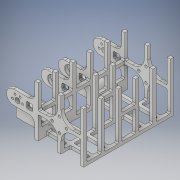
# Autodesk Inventor part: Double Holder V5
Saved by Autodesk Inventor 2019 (Build 230136000, 136)
## iProperties
Created: 2018-12-02
Part Number: Double Holder V5
Material: Generic
Document SubType Name: Modeling
Designer: Ashley
Density: 1 g/cm^3
Appearance: Default
Author: Ashley
Autodesk Inventor part; units mm, degrees
ref_plane "YZ Plane" through (0, 0, 0) normal (1, 0, 0) x (0, 1, 0)
ref_plane "XZ Plane" through (0, 0, 0) normal (0, 1, 0) x (-1, 0, 0)
ref_plane "XY Plane" through (0, 0, 0) normal (0, 0, 1) x (1, 0, 0)
sketch "Sketch1" plane through (0, 0, 0) normal (0, 1, 0) x (-1, 0, 0)
  line L0 (-40.25, -64) -> (40.25, -64) construction
  line L1 (40.25, -64) -> (40.25, 64) construction
  line L2 (40.25, 64) -> (-40.25, 64) construction
  line L3 (-40.25, 64) -> (-40.25, -64) construction
  line L4 (-40.25, -64) -> (40.25, 64) construction
  line L5 (40.25, -64) -> (-40.25, 64) construction
  line L6 (38.5, 71) -> (-38.5, 71) construction
  line L7 (-38.5, 71) -> (-38.5, 11) construction
  line L8 (-38.5, 11) -> (38.5, 11) construction
  line L9 (38.5, 11) -> (38.5, 71) construction
  line L10 (49.194, 0) -> (-57.7612, 0) construction
  line L11 (38.5, -71) -> (-38.5, -71) construction
  line L12 (-38.5, -71) -> (-38.5, -11) construction
  line L13 (-38.5, -11) -> (38.5, -11) construction
  line L14 (38.5, -11) -> (38.5, -71) construction
  line L15 (-38.5, -21) -> (-38.5, -31)
  line L16 (38.5, -31) -> (38.5, -21)
  line L17 (-38.5, -41) -> (-38.5, -51)
  line L18 (38.5, -51) -> (38.5, -41)
  line L19 (-38.5, 21) -> (-38.5, 31)
  line L20 (38.5, 31) -> (38.5, 21)
  line L21 (-38.5, 41) -> (-38.5, 51)
  line L22 (38.5, 51) -> (38.5, 41)
  line L23 (38.5, -11) -> (33.5, -11)
  line L24 (33.5, -71) -> (38.5, -71)
  line L25 (38.5, -71) -> (38.5, -11)
  line L26 (-38.5, -71) -> (-33.5, -71)
  line L27 (-33.5, -11) -> (-38.5, -11)
  line L28 (-38.5, -11) -> (-38.5, -71)
  line L29 (-38.5, 71) -> (-38.5, 11) construction
  line L30 (38.5, 11) -> (38.5, 71) construction
  line L31 (-38.5, 21) -> (-38.5, 31)
  line L32 (38.5, 31) -> (38.5, 21)
  line L33 (-38.5, 41) -> (-38.5, 51)
  line L34 (38.5, 51) -> (38.5, 41)
  line L35 (38.5, 11) -> (33.5, 11)
  line L36 (33.5, 71) -> (38.5, 71)
  line L37 (38.5, 71) -> (38.5, 11)
  line L38 (-38.5, 71) -> (-33.5, 71)
  line L39 (-33.5, 11) -> (-38.5, 11)
  line L40 (-38.5, 11) -> (-38.5, 71)
  line L41 (33.5, 11) -> (33.5, 26)
  line L42 (33.5, 31) -> (33.5, 51)
  line L43 (33.5, 56) -> (33.5, 71)
  line L44 (-33.5, 71) -> (-33.5, 56)
  line L45 (-33.5, 26) -> (-33.5, 11)
  line L46 (33.5, -11) -> (33.5, -26)
  line L47 (33.5, -31) -> (33.5, -51)
  line L48 (33.5, -56) -> (33.5, -71)
  line L49 (-33.5, -71) -> (-33.5, -56)
  line L50 (-33.5, -51) -> (-33.5, -31)
  line L51 (-33.5, -26) -> (-33.5, -11)
  line L52 (-33.5, 51) -> (-33.5, 31)
  line L53 (-2.5, -71) -> (2.5, -71)
  line L54 (2.5, 71) -> (-2.5, 71)
  line L55 (-2.5, -71) -> (2.5, 71) construction
  line L56 (2.5, -71) -> (-2.5, 71) construction
  line L57 (2.5, 56) -> (2.5, 71)
  line L58 (-33.5, 56) -> (-2.5, 56)
  line L59 (2.5, 56) -> (33.5, 56)
  line L60 (-2.5, 71) -> (-2.5, 56)
  line L61 (33.5, 51) -> (2.5, 51)
  line L62 (-2.5, 51) -> (-33.5, 51)
  line L63 (2.5, 31) -> (2.5, 51)
  line L64 (-33.5, 31) -> (-2.5, 31)
  line L65 (2.5, 31) -> (33.5, 31)
  line L66 (33.5, 26) -> (2.5, 26)
  line L67 (-2.5, 26) -> (-33.5, 26)
  line L68 (-2.5, 51) -> (-2.5, 31)
  line L69 (2.5, -26) -> (2.5, 26)
  line L70 (33.5, -26) -> (2.5, -26)
  line L71 (-2.5, -26) -> (-33.5, -26)
  line L72 (-33.5, -31) -> (-2.5, -31)
  line L73 (2.5, -31) -> (33.5, -31)
  line L74 (-2.5, 26) -> (-2.5, -26)
  line L75 (2.5, -71) -> (2.5, -56)
  line L76 (2.5, -51) -> (2.5, -31)
  line L77 (33.5, -51) -> (2.5, -51)
  line L78 (-2.5, -51) -> (-33.5, -51)
  line L79 (-33.5, -56) -> (-2.5, -56)
  line L80 (2.5, -56) -> (33.5, -56)
  line L81 (-2.5, -31) -> (-2.5, -51)
  line L82 (-2.5, -56) -> (-2.5, -71)
  point P0 (0, 0)
  dimension "d219" = 0
  dimension "d0" = 128
  dimension "d6" = 11
  dimension "d7" = 60
  dimension "d31" = 5
  dimension "d32" = 5
  dimension "d33" = 5
  dimension "d34" = 5
  dimension "d35" = 5
  dimension "d37" = 5
  dimension "d38" = 5
  dimension "d39" = 5
  dimension "d52" = 5
  dimension "d328" = 60
  dimension "d329" = 20
  dimension "d330" = 15
  dimension "d332" = 5
  dimension "d333" = 5
  dimension "d334" = 15
  dimension "d335" = 15
  dimension "d337" = 20
  dimension "d343" = 15
  dimension "d344" = 5
  dimension "d345" = 5
  dimension "d359" = 5
  dimension "d360" = 20
  dimension "d361" = 15
  dimension "d362" = 0
  dimension "d363" = 15
  dimension "d364" = 20
  dimension "d365" = 15
  dimension "d366" = 5
  dimension "d367" = 5
  dimension "d368" = 5
  dimension "d369" = 15
  dimension "d394" = 31
  dimension "d398" = 80.5
  dimension "d400" = 77
  dimension "d401" = 31
  dimension "d402" = 31
  dimension "d403" = 31
  dimension "d441" = 31
  dimension "d442" = 31
  dimension "d443" = 31
  dimension "d444" = 31
  dimension "d445" = 31
  dimension "d446" = 31
  dimension "d447" = 31
  dimension "d448" = 31
  constraints: 166 end point, 48 parallel, 20 symmetric about line, 19 perpendicular, 11 horizontal, 8 point on line, 6 midpoint
  measures "d0" distance of L0.end L1.end
  measures "d6" distance between parallel lines of L10 L8
  measures "d7" distance of L8.end L6.start
  measures "d31" distance between parallel lines of L9 L41
  measures "d32" distance between parallel lines of L9 L42
  measures "d33" distance between parallel lines of L9 L43
  measures "d34" distance between parallel lines of L14 L47
  measures "d35" distance between parallel lines of L12 L50
  measures "d37" distance between parallel lines of L7 L45
  measures "d38" distance between parallel lines of L7 L52
  measures "d39" distance between parallel lines of L7 L44
  measures "d52" distance of L54.end L54.start
  measures "d328" distance of L13.end L11.start
  measures "d329" distance between parallel lines of L62 L64
  measures "d330" distance between parallel lines of L67 L8
  measures "d332" distance between parallel lines of L58 L62
  measures "d333" distance between parallel lines of L64 L67
  measures "d334" distance between parallel lines of L6 L58
  measures "d335" distance between parallel lines of L8 L66
  measures "d337" distance between parallel lines of L61 L65
  measures "d343" distance between parallel lines of L6 L59
  measures "d344" distance between parallel lines of L65 L66
  measures "d345" distance between parallel lines of L59 L61
  measures "d359" distance between parallel lines of L77 L80
  measures "d360" distance between parallel lines of L73 L77
  measures "d361" distance between parallel lines of L11 L79
  measures "d362" distance between parallel lines of L11 L53
  measures "d363" distance between parallel lines of L11 L80
  measures "d364" distance between parallel lines of L72 L78
  measures "d365" distance between parallel lines of L13 L71
  measures "d366" distance between parallel lines of L79 L78
  measures "d367" distance between parallel lines of L70 L73
  measures "d368" distance between parallel lines of L71 L72
  measures "d369" distance between parallel lines of L13 L70
  measures "d394" distance between parallel lines of L63 L42
  measures "d398" distance between parallel lines of L3 L1
  measures "d400" distance between parallel lines of L9 L7
  measures "d401" distance between parallel lines of L68 L52
  measures "d402" distance between parallel lines of L81 L50
  measures "d403" distance between parallel lines of L47 L76
  measures "d441" distance between parallel lines of L43 L57
  measures "d442" distance between parallel lines of L44 L60
  measures "d443" distance between parallel lines of L69 L41
  measures "d444" distance between parallel lines of L45 L74
  measures "d445" distance between parallel lines of L46 L69
  measures "d446" distance between parallel lines of L51 L74
  measures "d447" distance between parallel lines of L75 L48
  measures "d448" distance between parallel lines of L49 L82
extrude "Base Extrusion" add sketch "Sketch1" along normal blind 5
sketch "Sketch4" plane through (0, 5, 0) normal (0, 1, 0) x (1, 0, 0)
  line L0 (-38.5, -71) -> (-33.5, -71)
  line L1 (-33.5, -71) -> (-33.5, -66)
  line L2 (-33.5, -66) -> (-38.5, -66)
  line L3 (-38.5, -66) -> (-38.5, -71)
  line L4 (-33.5, -11) -> (-38.5, -11)
  line L5 (-38.5, -11) -> (-38.5, -16)
  line L6 (-38.5, -16) -> (-33.5, -16)
  line L7 (-33.5, -16) -> (-33.5, -11)
  line L8 (2.5, -71) -> (-2.5, -71)
  line L9 (-2.5, -71) -> (-2.5, -66)
  line L10 (-2.5, -66) -> (2.5, -66)
  line L11 (2.5, -66) -> (2.5, -71)
  line L12 (33.5, -71) -> (38.5, -71)
  line L13 (38.5, -71) -> (38.5, -66)
  line L14 (38.5, -66) -> (33.5, -66)
  line L15 (33.5, -66) -> (33.5, -71)
  line L16 (38.5, -11) -> (33.5, -11)
  line L17 (33.5, -11) -> (33.5, -16)
  line L18 (33.5, -16) -> (38.5, -16)
  line L19 (38.5, -16) -> (38.5, -11)
  line L20 (38.5, -38.5) -> (33.5, -38.5)
  line L21 (33.5, -38.5) -> (33.5, -43.5)
  line L22 (33.5, -43.5) -> (38.5, -43.5)
  line L23 (38.5, -43.5) -> (38.5, -38.5)
  line L24 (38.5, -38.5) -> (33.5, -43.5) construction
  line L25 (33.5, -38.5) -> (38.5, -43.5) construction
  line L26 (2.5, -16) -> (-2.5, -16)
  line L27 (-2.5, -16) -> (-2.5, -11)
  line L28 (-2.5, -11) -> (2.5, -11)
  line L29 (2.5, -11) -> (2.5, -16)
  line L30 (2.5, -16) -> (-2.5, -11) construction
  line L31 (-2.5, -16) -> (2.5, -11) construction
  line L32 (-50.9334, 0) -> (57.8968, 0) construction
  line L33 (33.5, 71) -> (38.5, 71) construction
  line L34 (38.5, 11) -> (33.5, 11) construction
  line L35 (-33.5, 11) -> (-38.5, 11) construction
  line L36 (-38.5, 71) -> (-33.5, 71) construction
  line L37 (-38.5, 71) -> (-33.5, 71)
  line L38 (-33.5, 71) -> (-33.5, 66)
  line L39 (-33.5, 66) -> (-38.5, 66)
  line L40 (-38.5, 66) -> (-38.5, 71)
  line L41 (-33.5, 11) -> (-38.5, 11)
  line L42 (-38.5, 11) -> (-38.5, 16)
  line L43 (-38.5, 16) -> (-33.5, 16)
  line L44 (-33.5, 16) -> (-33.5, 11)
  line L45 (33.5, 71) -> (38.5, 71)
  line L46 (38.5, 71) -> (38.5, 66)
  line L47 (38.5, 66) -> (33.5, 66)
  line L48 (33.5, 66) -> (33.5, 71)
  line L49 (38.5, 11) -> (33.5, 11)
  line L50 (33.5, 11) -> (33.5, 16)
  line L51 (33.5, 16) -> (38.5, 16)
  line L52 (38.5, 16) -> (38.5, 11)
  line L53 (38.5, 38.5) -> (33.5, 38.5)
  line L54 (33.5, 38.5) -> (33.5, 43.5)
  line L55 (33.5, 43.5) -> (38.5, 43.5)
  line L56 (38.5, 43.5) -> (38.5, 38.5)
  line L57 (38.5, 38.5) -> (33.5, 43.5) construction
  line L58 (33.5, 38.5) -> (38.5, 43.5) construction
  line L59 (2.5, 16) -> (-2.5, 16)
  line L60 (-2.5, 16) -> (-2.5, 11)
  line L61 (-2.5, 11) -> (2.5, 11)
  line L62 (2.5, 11) -> (2.5, 16)
  line L63 (2.5, 16) -> (-2.5, 11) construction
  line L64 (-2.5, 16) -> (2.5, 11) construction
  line L65 (-33.5, 51) -> (-33.5, 31) construction
  line L66 (-38.5, 38.5) -> (-33.5, 38.5)
  line L67 (-33.5, 38.5) -> (-33.5, 43.5)
  line L68 (-33.5, 43.5) -> (-38.5, 43.5)
  line L69 (-38.5, 43.5) -> (-38.5, 38.5)
  line L70 (-38.5, 38.5) -> (-33.5, 43.5) construction
  line L71 (-33.5, 38.5) -> (-38.5, 43.5) construction
  line L72 (-38.5, -43.5) -> (-33.5, -43.5)
  line L73 (-33.5, -43.5) -> (-33.5, -38.5)
  line L74 (-33.5, -38.5) -> (-38.5, -38.5)
  line L75 (-38.5, -38.5) -> (-38.5, -43.5)
  line L76 (-38.5, -43.5) -> (-33.5, -38.5) construction
  line L77 (-33.5, -43.5) -> (-38.5, -38.5) construction
  line L78 (38.5, 71) -> (33.5, 71) construction
  line L79 (2.5, -71) -> (2.5, -56) construction
  line L80 (-2.5, 71) -> (2.5, 71)
  line L81 (2.5, 71) -> (2.5, 66)
  line L82 (2.5, 66) -> (-2.5, 66)
  line L83 (-2.5, 66) -> (-2.5, 71)
  line L84 (38.5, 11) -> (38.5, 71) construction
  line L85 (2.5, 56) -> (2.5, 71) construction
  line L86 (-33.5, -26) -> (-33.5, -11) construction
  line L87 (-38.5, -11) -> (-38.5, -71) construction
  point P0 (38.5, -71)
  point P1 (33.5, -11)
  point P2 (0, 0)
  point P3 (36, -41)
  point P4 (0, -13.5)
  point P5 (36, 41)
  point P6 (0, 13.5)
  point P7 (-36, 41)
  point P8 (-36, -41)
  dimension "d55" = 5
  dimension "d56" = 5
  dimension "d58" = 5
  dimension "d90" = 5
  dimension "d91" = 5
  dimension "d92" = 5
  dimension "d370" = 22.5
  dimension "d371" = 60
  dimension "d372" = 5
  dimension "d373" = 5
  dimension "d375" = 22.5
  dimension "d376" = 0
  dimension "d377" = 60
  dimension "d378" = 22.5
  dimension "d379" = 22.5
  dimension "d381" = 22.5
  dimension "d385" = 5
  dimension "d388" = 5
  dimension "d389" = 5
  dimension "d451" = 5
  dimension "d452" = 0
  dimension "d453" = 5
  dimension "d454" = 5
  dimension "d455" = 5
  dimension "d456" = 0
  dimension "d457" = 0
  dimension "d458" = 5
  dimension "d459" = 5
  dimension "d460" = 5
  dimension "d461" = 22.5
  dimension "d463" = 60
  dimension "d464" = 22.5
  dimension "d465" = 22.5
  constraints: 162 end point, 30 symmetric about line, 20 parallel, 12 midpoint, 11 horizontal, 10 perpendicular, 2 point on line
  measures "d55" distance of L1.end L0.end
  measures "d56" distance of L5.end L4.end
  measures "d58" distance of L21.end L20.end
  measures "d90" distance of L67.end L66.end
  measures "d91" distance of L74.end L73.end
  measures "d92" distance of L73.end L72.end
  measures "d370" distance between parallel lines of L51 L53
  measures "d371" distance between parallel lines of L34 L33
  measures "d372" distance between parallel lines of L53 L55
  measures "d373" distance between parallel lines of L47 L33
  measures "d375" distance between parallel lines of L47 L55
  measures "d376" distance between parallel lines of L45 L78
  measures "d377" distance of point (38.5, -71) L16.start
  measures "d378" distance between parallel lines of L14 L22
  measures "d379" distance between parallel lines of L20 L18
  measures "d381" distance between parallel lines of L39 L68
  measures "d385" distance between parallel lines of L9 L79
  measures "d388" distance of L81.end L82.end
  measures "d389" distance of L80.end L81.end
  measures "d451" distance between parallel lines of L48 L46
  measures "d452" distance between parallel lines of L84 L56
  measures "d453" distance between parallel lines of L54 L84
  measures "d454" distance between parallel lines of L52 L50
  measures "d455" distance between parallel lines of L34 L51
  measures "d456" distance between parallel lines of L85 L81
  measures "d457" distance between parallel lines of L87 L75
  measures "d458" distance between parallel lines of L3 L1
  measures "d459" distance between parallel lines of L86 L5
  measures "d460" distance between parallel lines of L67 L69
  measures "d461" distance between parallel lines of L43 L66
  measures "d463" distance of L87.start L0.start
  measures "d464" distance between parallel lines of L74 L6
  measures "d465" distance between parallel lines of L2 L72
extrude "Pegs Extrusions" add sketch "Sketch4" along normal blind 74.5
sketch "Sketch8" plane through (0, 5, 0) normal (0, 1, 0) x (1, 0, 0)
  line L0 (-38.5, 11) -> (-38.5, 71) construction
  line L1 (-33.5, 66) -> (-38.5, 66)
  line L2 (-38.5, 66) -> (-38.5, 16)
  line L3 (-38.5, 16) -> (-33.5, 16)
  line L4 (-33.5, 16) -> (-33.5, 66)
  line L5 (-38.5, -71) -> (-38.5, -11) construction
  line L6 (-38.5, -16) -> (-33.5, -16)
  line L7 (-33.5, -16) -> (-33.5, -66)
  line L8 (-33.5, -66) -> (-38.5, -66)
  line L9 (-38.5, -66) -> (-38.5, -16)
  line L10 (-33.5, -16) -> (-38.5, -16) projected
  line L11 (-38.5, -66) -> (-33.5, -66) projected
  line L12 (-33.5, 16) -> (-38.5, 16) construction
  line L13 (-38.5, 66) -> (-33.5, 66) construction
  point P0 (0, 0)
  dimension "d286" = 50
  dimension "d287" = 50
  dimension "d288" = 0
  dimension "d289" = 50
  dimension "d290" = 50
  dimension "d291" = 0
  dimension "d449" = 5
  dimension "d450" = 5
  constraints: 16 end point, 4 parallel, 2 horizontal, 2 perpendicular, 2 point on line
  measures "d286" distance between parallel lines of L8 L6
  measures "d287" distance between parallel lines of L11 L10
  measures "d288" distance between parallel lines of L6 L10
  measures "d289" distance between parallel lines of L12 L13
  measures "d290" distance between parallel lines of L3 L1
  measures "d291" distance between parallel lines of L13 L1
  measures "d449" distance between parallel lines of L0 L4
  measures "d450" distance between parallel lines of L5 L7
extrude "Front Extrusion" add sketch "Sketch8" along normal blind 11.5
sketch "Sketch9" plane through (-38.5, 0, 11) normal (-1, 0, 0) x (0, 0, 1)
  line L0 (11.5, 5) -> (48.5, 5) construction
  line L1 (8.0687, 8.5) -> (51.7383, 8.5) construction
  line L2 (9.6976, 12.5) -> (51.7383, 12.5) construction
  line L3 (43.5, 23.1119) -> (43.5, 2.014) construction
  line L4 (16.5, 23.1119) -> (16.5, 2.014) construction
  arc A0 (16.5, 12.5629) -> (43.5, 12.5629) centre (30, 32.9598) ccw
  line L5 (16.5, 12.5629) -> (16.5, 14.5629)
  line L6 (43.5, 12.5629) -> (43.5, 14.5629)
  arc A1 (16.5, 14.5629) -> (43.5, 14.5629) centre (30, 32.9598) ccw
  line L7 (60, 0) -> (60, 79.5) construction
  line L8 (-82, 0) -> (-82, 79.5) construction
  line L9 (32.5, 16.5) -> (32.5, 79.5) construction
  line L10 (27.5, 16.5) -> (27.5, 79.5) construction
  line L11 (5, 16.5) -> (5, 79.5) construction
  line L12 (55, 16.5) -> (55, 79.5) construction
  line L13 (0, 0) -> (0, 79.5) construction
  line L14 (-22, 0) -> (-22, 79.5) construction
  line L15 (-11, -14.5349) -> (-11, 42.196) construction
  line L16 (-33.5, 5) -> (-70.5, 5) construction
  line L17 (-30.0687, 8.5) -> (-73.7383, 8.5) construction
  line L18 (-31.6976, 12.5) -> (-73.7383, 12.5) construction
  line L19 (-65.5, 23.1119) -> (-65.5, 2.014) construction
  line L20 (-38.5, 23.1119) -> (-38.5, 2.014) construction
  arc A2 (-65.5, 12.5629) -> (-38.5, 12.5629) centre (-52, 32.9598) ccw
  line L21 (-38.5, 12.5629) -> (-38.5, 14.5629)
  line L22 (-65.5, 12.5629) -> (-65.5, 14.5629)
  arc A3 (-65.5, 14.5629) -> (-38.5, 14.5629) centre (-52, 32.9598) ccw
  dimension "d77" = 3.5
  dimension "d78" = 4
  dimension "d81" = 27
  dimension "d84" = 2
  dimension "d85" = 2
  dimension "d341" = 2.5
  dimension "d342" = 2.5
  dimension "d347" = 11.5
  dimension "d349" = 50
  dimension "d350" = 11.5
  dimension "d404" = 22
  dimension "d406" = 11
  constraints: 30 end point, 16 symmetric about line, 8 point on circle, 4 centre point, 4 point on line, 2 coincident, 2 horizontal, 2 midpoint, 2 vertical, 1 tangent, 2 other
  measures "d77" distance between parallel lines of L0 L1
  measures "d78" distance between parallel lines of L1 L2
  measures "d81" distance between parallel lines of L3 L4
  measures "d84" distance of L5.start L5.end
  measures "d85" distance of L6.start L6.end
  measures "d341" distance from line of A0.centre L10
  measures "d342" distance from line of L9 A0.centre
  measures "d347" distance between parallel lines of L4 L11
  measures "d349" distance between parallel lines of L12 L11
  measures "d350" distance between parallel lines of L12 L3
  measures "d404" distance between parallel lines of L13 L14
  measures "d406" distance between parallel lines of L13 L15
extrude "Tape MEasure Holes Sketch" cut sketch "Sketch9" against normal up to surface (5 mm away)
fillet "Fillet1" radius 0.5 2 edges at (-36, 14.5629, 27.5) (-36, 14.5629, 54.5)
fillet "Fillet2" radius 0.6 2 edges at (-36, 12.5629, 54.5) (-36, 12.5629, 27.5)
sketch "Sketch13" plane through (33.5, 0, 56) normal (-1, 0, 0) x (0, 0, 1)
  line L0 (15, 0) -> (0, 0) construction
  line L1 (10, 5) -> (10, 79.5) construction
  line L2 (10, 36.463) -> (15, 36.463)
  line L3 (15, 36.463) -> (15, 41.463)
  line L4 (15, 41.463) -> (10, 41.463)
  line L5 (10, 41.463) -> (10, 36.463)
  line L6 (-56, -4.0321) -> (-56, 65.3237) construction
  line L7 (-127, 0) -> (-127, 79.5) construction
  line L8 (-122, 5) -> (-122, 79.5) construction
  line L9 (-122, 36.463) -> (-127, 36.463)
  line L10 (-127, 36.463) -> (-127, 41.463)
  line L11 (-127, 41.463) -> (-122, 41.463)
  line L12 (-122, 41.463) -> (-122, 36.463)
  line L13 (-127, 0) -> (-127, 79.5) construction
  point P0 (15, 79.5)
  point P1 (-56, 0)
  dimension "d198" = 5
  dimension "d199" = 5
  dimension "d200" = 36.463
  dimension "d358" = 0
  constraints: 22 end point, 8 symmetric about line, 2 parallel, 2 point on line, 1 horizontal, 1 perpendicular, 1 vertical
  measures "d198" distance of L2.start L2.end
  measures "d199" distance between parallel lines of L2 L4
  measures "d200" distance between parallel lines of L0 L2
  measures "d358" distance between parallel lines of L13 L7
extrude "Side Reenforcements" add sketch "Sketch13" along normal blind 69.5
sketch "Sketch14" plane through (-38.5, 0, -71) normal (-1, 0, 0) x (0, 0, 1)
  line L0 (5, 16.5) -> (5, 79.5) construction
  line L1 (0, 0) -> (0, 79.5) construction
  line L2 (0, 51.663) -> (5, 51.663)
  line L3 (5, 51.663) -> (5, 29.463)
  line L4 (5, 29.463) -> (0, 29.463)
  line L5 (0, 29.463) -> (0, 51.663)
  line L6 (5, 41.463) -> (0, 41.463) construction
  line L7 (0, 41.463) -> (5, 41.463) construction
  line L8 (0, 36.463) -> (5, 36.463) construction
  line L9 (0, 36.463) -> (5, 36.463) construction
  line L10 (71, -9.8248) -> (71, 90.7022) construction
  line L11 (112, 28.863) -> (112, 84.0441) construction
  line L12 (-56, 28.863) -> (-56, 84.0441) construction
  arc A0 (16.5, 14.5629) -> (43.5, 14.5629) centre (30, 32.9598) ccw construction
  arc A1 (16.5, 12.5629) -> (43.5, 12.5629) centre (30, 32.9598) ccw construction
  line L13 (30, -7.2644) -> (30, 95.9334) construction
  line L14 (32.5, 16.5) -> (32.5, 79.5) construction
  line L15 (27.5, 16.5) -> (27.5, 79.5) construction
  line L16 (137, 16.5) -> (137, 79.5) construction
  line L17 (-11, -9.8248) -> (-11, 90.7022) construction
  line L18 (142, 51.663) -> (137, 51.663)
  line L19 (137, 51.663) -> (137, 29.463)
  line L20 (137, 29.463) -> (142, 29.463)
  line L21 (142, 29.463) -> (142, 51.663)
  line L22 (137, 41.463) -> (142, 41.463) construction
  line L23 (142, 41.463) -> (137, 41.463) construction
  line L24 (142, 36.463) -> (137, 36.463) construction
  line L25 (142, 36.463) -> (137, 36.463) construction
  line L26 (0, 79.5) -> (5, 79.5) construction
  line L27 (60, 0) -> (0, 0) construction
  line L28 (55, 79.5) -> (60, 79.5) construction
  line L29 (55, 5) -> (55, 79.5) construction
  line L30 (60, 0) -> (60, 79.5) construction
  line L31 (55, 49.663) -> (60, 49.663)
  line L32 (60, 49.663) -> (60, 28.263)
  line L33 (60, 28.263) -> (55, 28.263)
  line L34 (55, 28.263) -> (55, 49.663)
  line L35 (87, 5) -> (87, 79.5) construction
  line L36 (82, 0) -> (82, 79.5) construction
  line L37 (87, 49.663) -> (82, 49.663)
  line L38 (82, 49.663) -> (82, 28.263)
  line L39 (82, 28.263) -> (87, 28.263)
  line L40 (87, 28.263) -> (87, 49.663)
  point P0 (112, 32.9598)
  point P1 (112, 32.9598)
  dimension "d204" = 7
  dimension "d323" = 22.2
  dimension "d326" = 10.2
  dimension "d408" = 5
  dimension "d409" = 2.5
  dimension "d417" = 27.837
  dimension "d418" = 29.463
  dimension "d419" = 21.4
  dimension "d420" = 29.837
  dimension "d421" = 28.263
  constraints: 58 end point, 21 symmetric about line, 7 point on line, 4 parallel, 3 perpendicular, 2 horizontal, 2 vertical
  measures "d204" distance between parallel lines of L4 L8
  measures "d323" distance between parallel lines of L4 L2
  measures "d326" distance between parallel lines of L6 L2
  measures "d408" distance between parallel lines of L14 L15
  measures "d409" distance between parallel lines of L14 L13
  measures "d417" distance between parallel lines of L26 L2
  measures "d418" distance between parallel lines of L27 L4
  measures "d419" distance between parallel lines of L33 L31
  measures "d420" distance between parallel lines of L28 L31
  measures "d421" distance between parallel lines of L27 L33
extrude "Siding Extrusions" add sketch "Sketch14" along normal blind 45.1
sketch "Sketch17" plane through (38.5, 0, -71) normal (0, 0, -1) x (-1, 0, 0)
  circle A0 centre (104.5, 38.963) radius 4
  circle A1 centre (96.5363, 38.2017) radius 1.7
  circle A2 centre (112.4643, 38.2085) radius 1.7
  circle A3 centre (100.5, 45.8912) radius 1.7
  circle A4 centre (108.5, 45.8912) radius 1.7
  line L0 (117.906, 35.7017) -> (8.125, 35.7017) construction
  line L1 (100.5, 45.8912) -> (104.5, 38.963) construction
  line L2 (104.5, 38.963) -> (108.5, 45.8912) construction
  line L3 (77, 16.5) -> (77, 79.5) construction
  line L4 (77, 29.463) -> (122.1, 29.463) construction
  line L5 (77, 51.663) -> (122.1, 51.663) construction
  point P0 (38.5, 0)
  dimension "d306" = 8
  dimension "d307" = 3.4
  dimension "d308" = 3.4
  dimension "d309" = 8
  dimension "d310" = 8
  dimension "d311" = 3.4
  dimension "d312" = 3.4
  dimension "d313" = 8
  dimension "d314" = 8
  dimension "d315" = 60
  dimension "d316" = 60
  dimension "d321" = 27.5
  dimension "d324" = 22.2
  dimension "d325" = 12.7
  constraints: 6 end point, 5 centre point, 1 horizontal
  measures "d306" diameter of A0
  measures "d307" diameter of A1
  measures "d308" diameter of A2
  measures "d309" distance of L2.start A1.centre
  measures "d310" distance of A2.centre L2.start
  measures "d311" diameter of A3
  measures "d312" diameter of A4
  measures "d313" distance of L2.start L1.start
  measures "d314" distance of L2.start L2.end
  measures "d315" angle of L0 L1
  measures "d316" angle of L0 L2
  measures "d321" distance from line of L3 L2.start
  measures "d324" distance between parallel lines of L4 L5
  measures "d325" distance from line of L2.start L5
extrude "Motor Mounts" cut sketch "Sketch17" against normal up to surface (5 mm away)
sketch "Sketch16" plane through (-2.5, 5, -11) normal (0, 0, 1) x (1, 0, 0)
  line L0 (5, 0) -> (0, 0) construction
  line L1 (0, 74.5) -> (5, 74.5) construction
  line L2 (0, 0) -> (0, 74.5) construction
  line L3 (5, 0) -> (5, 74.5) construction
  line L4 (0, 39.75) -> (5, 39.75)
  line L5 (5, 39.75) -> (5, 34.75)
  line L6 (5, 34.75) -> (0, 34.75)
  line L7 (0, 34.75) -> (0, 39.75)
  line L8 (41, -5) -> (41, 74.5) construction
  line L9 (5, 0) -> (36, 0) construction
  line L10 (41, -5) -> (36, -5)
  line L11 (36, -5) -> (36, 0)
  line L12 (36, 0) -> (41, 0)
  line L13 (41, 0) -> (41, -5)
  line L14 (36, 34.75) -> (41, 34.75)
  line L15 (41, 34.75) -> (41, 39.75)
  line L16 (41, 39.75) -> (36, 39.75)
  line L17 (36, 39.75) -> (36, 34.75)
  line L18 (36, 34.75) -> (41, 39.75) construction
  line L19 (41, 34.75) -> (36, 39.75) construction
  line L20 (36, 74.5) -> (41, 74.5) construction
  line L21 (-31, -5) -> (-36, -5) construction
  line L22 (-36, -5) -> (-31, -5)
  line L23 (-31, -5) -> (-31, 0)
  line L24 (-31, 0) -> (-36, 0)
  line L25 (-36, 0) -> (-36, -5)
  point P0 (2.5, -5)
  point P1 (38.5, 37.25)
  dimension "d215" = 5
  dimension "d216" = 34.75
  dimension "d217" = 34.75
  dimension "d299" = 5
  dimension "d300" = 5
  dimension "d301" = 5
  dimension "d302" = 5
  dimension "d303" = 34.75
  dimension "d304" = 5
  dimension "d305" = 5
  dimension "d466" = 0
  constraints: 36 end point, 8 parallel, 4 horizontal, 4 perpendicular, 2 midpoint, 2 point on line
  measures "d215" distance of L4.end L5.end
  measures "d216" distance between parallel lines of L1 L4
  measures "d217" distance between parallel lines of L0 L6
  measures "d299" distance of L9.end L12.end
  measures "d300" distance of L10.end L9.end
  measures "d301" distance of L16.end L15.end
  measures "d302" distance of L15.end L14.end
  measures "d303" distance between parallel lines of L20 L16
  measures "d304" distance of L24.end L23.end
  measures "d305" distance of L23.end L22.end
  measures "d466" distance between parallel lines of L8 L15
extrude "Center Reenforcement" add sketch "Sketch16" along normal up to surface (22 mm away)
fillet "Fillet4" radius 10 8 edges at (-38.5, 51.663, -68.5) (-38.5, 29.463, -68.5) (-38.5, 29.463, 68.5) (-38.5, 51.663, 68.5) (-38.5, 49.663, -13.5) (-38.5, 49.663, 13.5) (-38.5, 28.263, 13.5) (-38.5, 28.263, -13.5)
fillet "Fillet6" radius 11.1 4 edges at (-83.6, 51.663, -68.5) (-83.6, 29.463, -68.5) (-83.6, 51.663, 68.5) (-83.6, 29.463, 68.5)
fillet "Fillet7" radius 19 8 edges at (-2.5, 41.463, 68.5) (2.5, 41.463, 68.5) (-2.5, 36.463, 68.5) (2.5, 36.463, 68.5) (2.5, 36.463, -68.5) (-2.5, 36.463, -68.5) (2.5, 41.463, -68.5) (-2.5, 41.463, -68.5)
sketch "Sketch18" plane through (38.5, 0, 71) normal (0, 0, 1) x (1, 0, 0)
  circle A0 centre (-27.1863, 38.963) radius 2.1
  circle A1 centre (-38.5, 50.2767) radius 2.1
  circle A2 centre (-49.8137, 38.963) radius 2.1
  circle A3 centre (-38.5, 27.6493) radius 2.1
  point P0 (-38.5, 0)
  dimension "d264" = 4.2
  dimension "d267" = 4.2
  dimension "d270" = 4.2
  dimension "d271" = 4.2
  constraints: 4 centre point
  measures "d264" diameter of A0
  measures "d267" diameter of A1
  measures "d270" diameter of A2
  measures "d271" diameter of A3
extrude "Hub Mount" cut sketch "Sketch18" against normal up to surface (5 mm away)
mirror "Mirror1" about plane through (0, 0, 0) normal (0, 0, 1) of "Hub Mount"
sketch "Sketch22" plane through (-48.5, 49.663, -16) normal (0, 0, -1) x (-1, 0, 0)
  line L0 (35.1, 0) -> (35.1, -21.4) construction
  line L1 (0, 0) -> (35.1, 0) construction
  circle A0 centre (17.5, -10.7) radius 4 construction
  circle A1 centre (17.5, -10.7) radius 4 construction
  circle A2 centre (17.5, -10.7) radius 7.25
  line L2 (32.6, 0) -> (35.1, 0)
  line L3 (35.1, 0) -> (35.1, -21.4)
  line L4 (35.1, -21.4) -> (32.6, -21.4)
  line L5 (32.6, -21.4) -> (32.6, 0)
  point P0 (-48.5, -49.663)
  point P1 (-8.75, 0)
  dimension "d435" = 14.5
  dimension "d436" = 2.5
  constraints: 8 end point, 2 centre point, 2 coincident, 2 parallel, 1 horizontal, 1 perpendicular, 1 point on line
  measures "d435" diameter of A2
  measures "d436" distance between parallel lines of L0 L5
extrude "Axel Hole" cut sketch "Sketch22" against normal up to surface (32 mm away) contours A2
mirror "Mirror2" about plane through (0, 0, 0) normal (0, 0, 1) of "Motor Mounts"
sketch "Sketch26" plane through (38.5, 5, -66) normal (0, 0, 1) x (1, 0, 0)
  line L0 (-72, 31.5085) -> (-77, 31.5085)
  line L1 (-77, 31.5085) -> (-77, 36.5085)
  line L2 (-77, 36.5085) -> (-72, 36.5085)
  line L3 (-72, 36.5085) -> (-72, 31.5085)
  point P0 (-38.5, -5)
  dimension "d540" = 5
  dimension "d541" = 5
  constraints: 8 end point, 2 parallel, 1 horizontal, 1 perpendicular
  measures "d540" distance of L1.end L2.end
  measures "d541" distance of L0.end L1.end
extrude "Extrusion23" add sketch "Sketch26" along normal up to surface (132 mm away)
fillet "Fillet21" radius 10.7 4 edges at (-83.6, 49.663, -13.5) (-83.6, 28.263, -13.5) (-83.6, 49.663, 13.5) (-83.6, 28.263, 13.5)
sketch "Sketch23" plane through (-38.5, 32.9598, -41) normal (-1, 0, 0) x (0, 0, 1)
  line L0 (13.5, -18.3968) -> (13.5, -20.3968) construction
  arc A0 (-13.5, -20.3968) -> (13.5, -20.3968) centre (0, 0) ccw construction
  line L1 (-13.5, -20.3968) -> (-13.5, -18.3968) construction
  arc A1 (-13.5, -20.3968) -> (13.5, -20.3968) centre (0, 0) ccw
  line L2 (-11.1847, 0) -> (9.448, 0) construction
  line L3 (-13.5, -18.3968) -> (-13.5, -18.3968) construction
  line L4 (-13.5, -20.3968) -> (-13.5, -18.3968)
  line L5 (-14.626, -22.0982) -> (-14.626, -18.3968)
  line L6 (-14.626, -18.3968) -> (-13.5, -18.3968)
  line L7 (14.626, -22.0982) -> (14.626, -18.3968)
  line L8 (13.5, -18.3968) -> (13.5, -18.3968) construction
  line L9 (13.5, -18.3968) -> (14.626, -18.3968)
  line L10 (13.5, -20.3968) -> (13.5, -18.3968) construction
  line L11 (13.5, -20.3968) -> (13.5, -18.3968)
  line L12 (-12.5, -32.9598) -> (-9, -32.9598) construction
  line L13 (-16, -32.9598) -> (-12.5, -32.9598) construction
  line L14 (-13.126, -23.0208) -> (-13.126, -32.9598)
  line L15 (-13.126, -32.9598) -> (-14.626, -32.9598)
  line L16 (-14.626, -32.9598) -> (-14.626, -21.2098)
  line L17 (-8.5007, -25.0996) -> (-8.5007, -32.9598)
  line L18 (-8.5007, -32.9598) -> (-10.0007, -32.9598)
  line L19 (-10.0007, -32.9598) -> (-10.0007, -24.5405)
  line L20 (-3.8753, -26.2151) -> (-3.8753, -32.9598)
  line L21 (-3.8753, -32.9598) -> (-5.3753, -32.9598)
  line L22 (-5.3753, -32.9598) -> (-5.3753, -25.9491)
  line L23 (0.75, -26.4894) -> (0.75, -32.9598)
  line L24 (0.75, -32.9598) -> (-0.75, -32.9598)
  line L25 (-0.75, -32.9598) -> (-0.75, -26.4894)
  line L26 (5.3753, -25.9491) -> (5.3753, -32.9598)
  line L27 (5.3753, -32.9598) -> (3.8753, -32.9598)
  line L28 (3.8753, -32.9598) -> (3.8753, -26.2151)
  line L29 (10.0007, -24.5405) -> (10.0007, -32.9598)
  line L30 (10.0007, -32.9598) -> (8.5007, -32.9598)
  line L31 (8.5007, -32.9598) -> (8.5007, -25.0996)
  line L32 (12.5, -32.9598) -> (16, -32.9598) construction
  line L33 (13.126, -23.0208) -> (13.126, -32.9598)
  line L34 (13.126, -32.9598) -> (14.626, -32.9598)
  line L35 (14.626, -32.9598) -> (14.626, -21.0003)
  arc A2 (10.0007, -24.5405) -> (13.126, -23.0208) centre (0, 0) ccw
  arc A3 (5.3753, -25.9491) -> (8.5007, -25.0996) centre (0, 0) ccw
  arc A4 (0.75, -26.4894) -> (3.8753, -26.2151) centre (0, 0) ccw
  arc A5 (-3.8753, -26.2151) -> (-0.75, -26.4894) centre (0, 0) ccw
  arc A6 (-13.126, -23.0208) -> (-10.0007, -24.5405) centre (0, 0) ccw
  arc A7 (-8.5007, -25.0996) -> (-5.3753, -25.9491) centre (0, 0) ccw
  line L36 (41, -48.649) -> (41, -1.2234) construction
  line L37 (51, -30.4598) -> (109.5, -30.4598) construction
  line L38 (68.5, -18.3968) -> (58, -18.9598) construction
  line L39 (68.5, -18.3968) -> (68.5, -20.3968) construction
  arc A8 (68.5, -20.3968) -> (95.5, -20.3968) centre (82, 0) ccw construction
  line L40 (95.5, -20.3968) -> (95.5, -18.3968) construction
  line L41 (106, -18.9598) -> (95.5, -18.3968) construction
  arc A9 (68.5, -20.3968) -> (95.5, -20.3968) centre (82, 0) ccw
  line L42 (95.5, -18.3968) -> (95.5, -18.3968) construction
  line L43 (95.5, -20.3968) -> (95.5, -18.3968)
  line L44 (96.626, -22.0982) -> (96.626, -18.3968)
  line L45 (96.626, -18.3968) -> (95.5, -18.3968)
  line L46 (67.374, -22.0982) -> (67.374, -18.3968)
  line L47 (68.5, -18.3968) -> (68.5, -18.3968) construction
  line L48 (68.5, -18.3968) -> (67.374, -18.3968)
  line L49 (68.5, -20.3968) -> (68.5, -18.3968) construction
  line L50 (68.5, -20.3968) -> (68.5, -18.3968)
  line L51 (94.5, -32.9598) -> (91, -32.9598) construction
  line L52 (98, -32.9598) -> (94.5, -32.9598) construction
  line L53 (95.126, -23.0208) -> (95.126, -32.9598)
  line L54 (95.126, -32.9598) -> (96.626, -32.9598)
  line L55 (96.626, -32.9598) -> (96.626, -21.2098)
  line L56 (90.5007, -25.0996) -> (90.5007, -32.9598)
  line L57 (90.5007, -32.9598) -> (92.0007, -32.9598)
  line L58 (92.0007, -32.9598) -> (92.0007, -24.5405)
  line L59 (111, -32.9598) -> (-29, -32.9598) construction
  line L60 (85.8753, -26.2151) -> (85.8753, -32.9598)
  line L61 (85.8753, -32.9598) -> (87.3753, -32.9598)
  line L62 (87.3753, -32.9598) -> (87.3753, -25.9491)
  line L63 (81.25, -26.4894) -> (81.25, -32.9598)
  line L64 (81.25, -32.9598) -> (82.75, -32.9598)
  line L65 (82.75, -32.9598) -> (82.75, -26.4894)
  line L66 (76.6247, -25.9491) -> (76.6247, -32.9598)
  line L67 (76.6247, -32.9598) -> (78.1247, -32.9598)
  line L68 (78.1247, -32.9598) -> (78.1247, -26.2151)
  line L69 (71.9993, -24.5405) -> (71.9993, -32.9598)
  line L70 (71.9993, -32.9598) -> (73.4993, -32.9598)
  line L71 (73.4993, -32.9598) -> (73.4993, -25.0996)
  line L72 (69.5, -32.9598) -> (66, -32.9598) construction
  line L73 (68.874, -23.0208) -> (68.874, -32.9598)
  line L74 (68.874, -32.9598) -> (67.374, -32.9598)
  line L75 (67.374, -32.9598) -> (67.374, -21.0003)
  arc A10 (68.874, -23.0208) -> (71.9993, -24.5405) centre (82, 0) ccw
  arc A11 (73.4993, -25.0996) -> (76.6247, -25.9491) centre (82, 0) ccw
  arc A12 (78.1247, -26.2151) -> (81.25, -26.4894) centre (82, 0) ccw
  arc A13 (82.75, -26.4894) -> (85.8753, -26.2151) centre (82, 0) ccw
  arc A14 (92.0007, -24.5405) -> (95.126, -23.0208) centre (82, 0) ccw
  arc A15 (87.3753, -25.9491) -> (90.5007, -25.0996) centre (82, 0) ccw
  point P0 (31, -30.4598)
  point P1 (-24, -18.9598)
  point P2 (41, -32.9598)
  point P3 (111, -32.9598)
  point P4 (0.75, -26.4894)
  point P5 (81.25, -26.4894)
  dimension "d468" = 24.4598
  dimension "d469" = 66.999
  dimension "d471" = 1.126
  dimension "d472" = 1.126
  dimension "d474" = 1.5
  dimension "d475" = 1.5
  dimension "d477" = 1.5
  dimension "d479" = 1.5
  dimension "d481" = 1.5
  dimension "d483" = 1.5
  dimension "d485" = 1.5
  dimension "d486" = 3.1254
  dimension "d487" = 3.1254
  dimension "d488" = 3.1254
  dimension "d489" = 3.1254
  dimension "d490" = 29.2521
  dimension "d491" = 3.1254
  dimension "d492" = 3.1254
  dimension "d493" = 14.5629
  dimension "d495" = 70
  constraints: 138 end point, 59 symmetric about line, 32 point on circle, 28 coincident, 15 centre point, 10 point on line, 7 parallel, 4 vertical, 1 horizontal, 1 perpendicular, 15 other
  measures "d468" radius of A0
  measures "d471" distance between parallel lines of L1 L5
  measures "d472" distance between parallel lines of L7 L0
  measures "d474" distance of L14.end L15.end
  measures "d475" distance of L17.end L18.end
  measures "d477" distance of L20.end L21.end
  measures "d479" distance of L23.end L24.end
  measures "d481" distance of L26.end L27.end
  measures "d483" distance of L29.end L30.end
  measures "d485" distance of L34.end L33.end
  measures "d486" distance between parallel lines of L19 L14
  measures "d487" distance between parallel lines of L22 L17
  measures "d488" distance between parallel lines of L25 L20
  measures "d489" distance between parallel lines of L28 L23
  measures "d490" distance between parallel lines of L35 L16
  measures "d491" distance between parallel lines of L31 L26
  measures "d492" distance between parallel lines of L33 L29
  measures "d493" distance between parallel lines of L13 L6
  measures "d495" distance from line of point (111, -32.96) L36
extrude "Extrusion20" add sketch "Sketch23" along normal blind 45
ref_plane "Work Plane7" through (-72.5, 49.163, 71) normal (0, 0, 1) x (1, 0, 0)
sketch "Sketch24" plane through (-72.5, 49.163, 71) normal (0, 0, 1) x (1, 0, 0)
  line L0 (20.5, -3.6) -> (30.5, -3.6)
  line L1 (30.5, -3.6) -> (30.5, -13.6)
  line L2 (30.5, -13.6) -> (20.5, -13.6)
  line L3 (20.5, -13.6) -> (20.5, -3.6)
  point P0 (72.5, -49.163)
  dimension "d520" = 10
  dimension "d521" = 10
  constraints: 8 end point, 2 parallel, 1 horizontal, 1 perpendicular
  measures "d520" distance of L0.end L1.end
  measures "d521" distance of L0.start L0.end
extrude "Extrusion21" cut sketch "Sketch24" against normal up to surface (5 mm away)
ref_plane "Work Plane6" through (-72.9, 47.163, 16) normal (0, 0, 1) x (1, 0, 0)
sketch "Sketch25" plane through (-72.9, 47.163, 16) normal (0, 0, 1) x (1, 0, 0)
  line L0 (32.0845, -13.2) -> (22.0845, -13.2)
  line L1 (22.0845, -13.2) -> (22.0845, -3.2)
  line L2 (22.0845, -3.2) -> (32.0845, -3.2)
  line L3 (32.0845, -3.2) -> (32.0845, -13.2)
  line L4 (32.0845, -13.2) -> (22.0845, -3.2) construction
  line L5 (22.0845, -13.2) -> (32.0845, -3.2) construction
  point P0 (72.9, -47.163)
  point P1 (27.0845, -8.2)
  dimension "d528" = 10
  dimension "d529" = 10
  constraints: 12 end point, 2 midpoint, 2 parallel, 1 horizontal, 1 perpendicular
  measures "d528" distance of L1.end L2.end
  measures "d529" distance of L0.end L1.end
extrude "Extrusion22" cut sketch "Sketch25" against normal up to surface (5 mm away)
fillet "Fillet25" radius 0.5 4 edges at (-58.75, 38.963, 11) (-58.75, 38.963, 16) (-58.75, 38.963, -11) (-58.75, 38.963, -16)
fillet "Fillet27" radius 2 65 edges at (0, 5, 66) (36, 5, 66) (-33.5, 5, 53.5) (-33.5, 5, 28.5) (0, 5, 11) (0, 44.75, 11) (36, 44.75, 11) (36, 5, 38.5) (36, 5, 11) (36, 5, -16) (36, 5, -43.5) (0, 5, -16) (-33.5, 5, -28.5) (-33.5, 5, -53.5) (0, 5, -66) (0, 44.75, -11) (36, 44.75, -11) (36, 5, -66) (36, 5, -38.5) (36, 5, -11) (0, 5, -11) (36, 5, 16) (36, 5, 43.5) (0, 5, 16) (0, 39.75, -11) (36, 39.75, -11) (-36, 36.5085, -66) (-36, 36.5085, -38.5) (-36, 36.5085, -11) (-36, 36.5085, 16) (-36, 36.5085, 43.5) (-36, 16.5, 43.5) (-36, 16.5, 16) (-36, 16.5, -38.5) (-36, 16.5, -66) (-36, 41.5085, -38.5) (-36, 41.5085, -11) (-36, 41.5085, 16) (-36, 41.5085, 43.5) (36, 39.75, 11) (0, 39.75, 11) (-36, 36.5085, 11) (-36, 36.5085, 38.5) (-36, 36.5085, 66) (-36, 36.5085, -16) (-36, 36.5085, -43.5) (-33.5, 36.463, -68.5) (-33.5, 41.463, -68.5) (33.5, 36.463, -68.5) (33.5, 41.463, -68.5) (33.5, 41.463, 68.5) (33.5, 36.463, 68.5) (-33.5, 36.463, 68.5) (-33.5, 41.463, 68.5) (-36, 41.5085, 66) (-36, 16.5, 66) (-36, 16.5, 38.5) (-36, 16.5, -16) (-36, 16.5, -43.5) (-36, 41.5085, -43.5) (-36, 41.5085, -16) (-36, 41.5085, 11) (-36, 5, 11) (-36, 5, -11) (-36, 41.5085, 38.5)
fillet "Fillet28" radius 2 30 edges at (2.5, 2.5, 56) (-33.5, 3.5, 56) (-2.5, 2.5, 56) (-33.5, 3.5, 51) (-33.5, 3.5, 26) (-33.5, 3.5, 31) (-2.5, 2.5, 51) (-2.5, 2.5, 31) (2.5, 2.5, 31) (2.5, 2.5, -26) (33.5, 2.5, 26) (33.5, 2.5, 51) (2.5, 2.5, 51) (33.5, 2.5, 31) (2.5, 2.5, 26) (33.5, 2.5, -26) (-2.5, 2.5, 26) (-2.5, 2.5, -26) (-33.5, 3.5, -26) (2.5, 2.5, -51) (-33.5, 3.5, -51) (-33.5, 3.5, -31) (-2.5, 2.5, -31) (33.5, 2.5, -51) (33.5, 2.5, -31) (2.5, 2.5, -31) (-40.8155, 33.963, 13.5) (-40.8155, 43.963, 13.5) (-50.8155, 33.963, 13.5) (-50.8155, 43.963, 13.5)
ref_plane "Work Plane8" through (-38.5, 79.5, 0) normal (0, 0, 1) x (1, 0, 0)
mirror "Mirror4" about plane through (-38.5, 79.5, 0) normal (0, 0, 1) of "Extrusion22", "Extrusion21"
fillet "Fillet29" radius 2 12 edges at (-42, 35.563, 68.5) (-52, 35.563, 68.5) (-52, 45.563, 68.5) (-42, 45.563, 68.5) (-42, 45.563, -68.5) (-52, 45.563, -68.5) (-42, 35.563, -68.5) (-52, 35.563, -68.5) (-40.8155, 33.963, -13.5) (-50.8155, 33.963, -13.5) (-50.8155, 43.963, -13.5) (-40.8155, 43.963, -13.5)
fillet "Fillet30" radius 2 7 edges at (-38.5, 39.0085, 16) (-38.5, 39.0085, 66) (-38.5, 39.0085, 11) (-38.5, 39.0085, -16) (-38.5, 39.0085, -11) (-38.5, 38.0085, -66) (-33.5, 38.9858, 66)
fillet "Fillet31" radius 2 1 edges at (-37, 41.5085, -66)
fillet "Fillet32" radius 2 5 edges at (-33.5, 3.5, -56) (-2.5, 2.5, -56) (2.5, 2.5, -56) (33.5, 2.5, -56) (-2.5, 2.5, -51)
body "Solid1"
